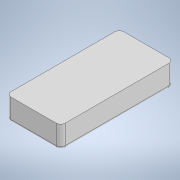
# Autodesk Inventor part: rasberry pi
Saved by Autodesk Inventor 2020 (Build 240168000, 168)
## iProperties
Created: 2019-09-04
Part Number: rasberry pi
Material: Generic
Document SubType Name: Modeling
Designer: User
Density: 1 g/cm^3
Appearance: Default
Author: User
Autodesk Inventor part; units mm, degrees
ref_plane "YZ Plane" through (0, 0, 0) normal (1, 0, 0) x (0, 1, 0)
ref_plane "XZ Plane" through (0, 0, 0) normal (0, 1, 0) x (-1, 0, 0)
ref_plane "XY Plane" through (0, 0, 0) normal (0, 0, 1) x (1, 0, 0)
sketch "Sketch1" plane through (0, 0, 0) normal (0, 1, 0) x (-1, 0, 0)
  line L0 (-19.05, 39.5605) -> (19.05, 39.5605)
  line L1 (19.05, 39.5605) -> (19.05, -39.5605)
  line L2 (19.05, -39.5605) -> (-19.05, -39.5605)
  line L3 (-19.05, -39.5605) -> (-19.05, 39.5605)
  line L4 (-19.05, 39.5605) -> (19.05, -39.5605) construction
  line L5 (19.05, 39.5605) -> (-19.05, -39.5605) construction
  point P0 (0, 0)
  dimension "d0" = 79.121
  dimension "d1" = 38.1
  constraints: 12 end point, 2 midpoint, 2 parallel, 1 horizontal, 1 perpendicular
  measures "d0" distance of L0.end L1.end
  measures "d1" distance between parallel lines of L3 L1
extrude "Extrusion1" add sketch "Sketch1" along normal blind 15.24
fillet "Fillet1" radius 1.5875 4 edges at (19.05, 0, 0) (0, 0, 39.5605) (-19.05, 0, 0) (0, 0, -39.5605)
fillet "Fillet1" radius 3.175 4 edges at (-19.05, 7.62, -39.5605) (19.05, 7.62, -39.5605) (19.05, 7.62, 39.5605) (-19.05, 7.62, 39.5605)
body "Solid1"
